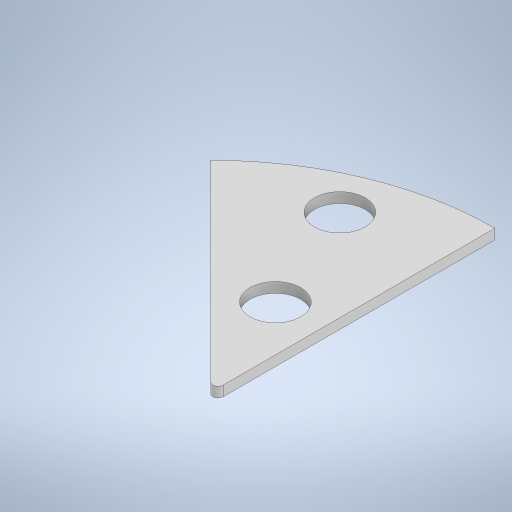
# Autodesk Inventor part: Todd
Saved by Autodesk Inventor 2023 (Build 270158000, 158)
## iProperties
Created: 2023-01-31
Part Number: Todd
Material: Generic
Document SubType Name: Modeling
Designer: Gabriel - T3 CAD
Density: 1 g/cm^3
Appearance: Default
Author: Gabriel - T3 CAD
Autodesk Inventor part; units mm, degrees
ref_plane "YZ Plane" through (0, 0, 0) normal (1, 0, 0) x (0, 1, 0)
ref_plane "XZ Plane" through (0, 0, 0) normal (0, 1, 0) x (-1, 0, 0)
ref_plane "XY Plane" through (0, 0, 0) normal (0, 0, 1) x (1, 0, 0)
sketch "Sketch1" plane through (0, 0, 0) normal (0, 1, 0) x (-1, 0, 0)
  circle A0 centre (0, 0) radius 177.8
  line L0 (0, 0) -> (0, -177.8)
  line L1 (0, 0) -> (177.8, 0) construction
  line L2 (0, 0) -> (125.7236, -125.7236)
  line L3 (0, 0) -> (177.8, 0) construction
  circle A1 centre (28.575, -68.9862) radius 15.875
  circle A2 centre (57.1059, -137.8659) radius 15.875
  line L4 (0, 0) -> (68.0411, -164.2658)
  line L5 (0, 0) -> (177.8, 0) construction
  dimension "d0" = 355.6
  dimension "d1" = 177.8
  dimension "d2" = 90
  dimension "d3" = 177.8
  dimension "d4" = 45
  dimension "d8" = 31.75
  dimension "d9" = 177.8
  dimension "d10" = 67.5
  dimension "d11" = 28.575
  dimension "d12" = 149.225
  constraints: 12 end point, 3 centre point, 3 equal length, 3 horizontal, 2 point on line, 1 coincident, 1 equal radius
  measures "d0" diameter of A0
  measures "d1" distance of L0.start L0.end
  measures "d2" angle of L0 L1
  measures "d3" distance of L0.start L2.end
  measures "d4" angle of L2 L3
  measures "d8" diameter of A2
  measures "d9" distance of L0.start L4.end
  measures "d10" angle of L4 L5
  measures "d11" distance from line of A1.centre L2
  measures "d12" distance of L0.start A2.centre
extrude "Extrusion1" add sketch "Sketch1" along normal blind 6.35 contours L0 L4 A1 A2 A0 | A0 L4 A2 A1 L2
fillet "Fillet1" radius 3.175 1 edges at (0, 3.175, 0)
body "Solid1"
